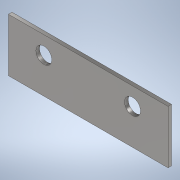
# Autodesk Inventor part: Plate B connector box-iv stand
Saved by Autodesk Inventor 2020 (Build 240168000, 168)
## iProperties
Created: 2020-07-06
Part Number: Plate B connector box-iv stand
Material: Steel, Carbon
Document SubType Name: Sheet Metal
Designer: Bruno
Density: 7.85 g/cm^3
Sheet Metal Rule: Default_mm
Appearance: Semi-Polished
Author: Bruno
Autodesk Inventor part; units mm, degrees
ref_plane "YZ Plane" through (0, 0, 0) normal (1, 0, 0) x (0, 1, 0)
ref_plane "XZ Plane" through (0, 0, 0) normal (0, 1, 0) x (-1, 0, 0)
ref_plane "XY Plane" through (0, 0, 0) normal (0, 0, 1) x (1, 0, 0)
sketch "Sketch1" plane through (0, 0, 0) normal (0, 0, 1) x (1, 0, 0)
  line L0 (0, -3.4) -> (45, -3.4)
  line L1 (45, -3.4) -> (45, 11.6)
  line L2 (45, 11.6) -> (0, 11.6)
  line L3 (0, 11.6) -> (0, -3.4)
  point P0 (0, 0)
  dimension "d1" = 3.4
  dimension "d2" = 45
  dimension "d3" = 45
  dimension "d4" = 15
  measures "d1" vertical distance of point (0, 0) point (45, -3.4)
  measures "d2" horizontal distance of point (0, 0) point (45, -3.4)
  measures "d3" distance of L2.end L1.end
  measures "d4" distance of L1.end L0.end
extrude "Plate1" add sketch "Sketch1" along normal blind 1
sketch "Sketch2" plane through (0, 0, 1) normal (0, 0, 1) x (1, 0, 0)
  line L0 (45, -3.4) -> (0, -3.4) projected
  line L1 (45, 11.6) -> (45, -3.4) projected
  line L2 (0, -3.4) -> (0, 11.6) projected
  point P0 (0, 0)
  point P1 (35, 6.6)
  point P2 (10, 6.6)
  dimension "d5" = 10
  dimension "d6" = 10
  dimension "d7" = 10
  constraints: 1 horizontal alignment
  measures "d5" distance from line of L0 point (35, 6.6)
  measures "d6" distance from line of point (35, 6.6) L1
  measures "d7" distance from line of L2 point (10, 6.6)
hole "Hole1" at (35, 6.6, 1) at (10, 6.6, 1) direction (0, 0, -1) diameter 4.5 end through all
equation "\"d13\" = Thickness"
equation "\"d0\" = Thickness"
equation "\"BendRadius\" = Thickness"
equation "\"BendReliefWidth\" = Thickness"
equation "\"BendReliefDepth\" = 0.5 * Thickness"
equation "\"CornerReliefSize\" = 4 * Thickness"
equation "\"MinimumRemnant\" = 2 * Thickness"
equation "\"TransitionRadius\" = BendRadius"
equation "\"JacobiRadiusSize\" = BendRadius"
equation "\"GapSize\" = Thickness"
equation "\"Thickness\" = 1"
body "Solid1"
